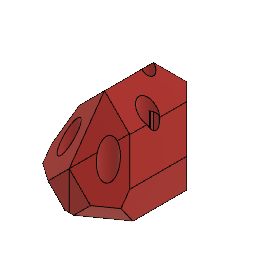
ender_sw_stealth_idler (Autodesk Fusion 360 design; units mm, degrees)
Autodesk Fusion 360 part; units mm, degrees
sketch "Sketch1" plane through (0, 0, 0) normal (0, 0, 1) x (1, 0, 0)
  line L0 (0, 0) -> (-1, 0) construction
  line L1 (-1, 0) -> (-41, 0)
  line L2 (-41, 0) -> (-41, 60)
  line L3 (-41, 60) -> (-1, 60)
  line L4 (-1, 60) -> (-1, 0)
  line L5 (-1, 0) -> (-21, 0) construction
  line L6 (-21, 0) -> (-21, 65.8302) construction
  line L7 (-1, 0) -> (-1, 20) construction
  line L8 (-1, 20) -> (-78.7718, 20) construction
  line L9 (-21, 0) -> (-21, 10) construction
  line L10 (-21, 10) -> (-11, 10) construction
  circle A0 centre (-11, 10) radius 2.55
  circle A1 centre (-11, 30) radius 2.55
  circle A2 centre (-31, 10) radius 2.55
  circle A3 centre (-31, 30) radius 2.55
  line L11 (-21, 20) -> (-21, 30) construction
  line L12 (-16, 35) -> (-26, 35)
  line L13 (-26, 35) -> (-26, 25)
  line L14 (-26, 25) -> (-16, 25)
  line L15 (-16, 25) -> (-16, 35)
  line L16 (-16, 35) -> (-26, 25) construction
  line L17 (-26, 35) -> (-16, 25) construction
  line L18 (-21, 30) -> (-21, 40) construction
  line L19 (-8.75, 46.5) -> (-33.25, 46.5)
  line L20 (-33.25, 46.5) -> (-33.25, 33.5)
  line L21 (-33.25, 33.5) -> (-8.75, 33.5)
  line L22 (-8.75, 33.5) -> (-8.75, 46.5)
  line L23 (-8.75, 46.5) -> (-33.25, 33.5) construction
  line L24 (-33.25, 46.5) -> (-8.75, 33.5) construction
  line L25 (-26, 48) -> (-16, 48)
  line L26 (-16, 48) -> (-16, 45)
  line L27 (-16, 45) -> (-26, 45)
  line L28 (-26, 45) -> (-26, 48)
  line L29 (-26, 48) -> (-16, 45) construction
  line L30 (-16, 48) -> (-26, 45) construction
  circle A4 centre (-21, 40) radius 1.55
  point P0 (-21, 30)
  point P1 (-21, 40)
  point P2 (-21, 46.5)
  dimension "d1" = 1
  dimension "d2" = 40
  dimension "d3" = 60
  dimension "d4" = 20
  dimension "d5" = 20
  dimension "d6" = 10
  dimension "d7" = 10
  dimension "d8" = 5.1
  dimension "d12" = 10
  dimension "d13" = 10
  dimension "d14" = 10
  dimension "d15" = 10
  dimension "d16" = 24.5
  dimension "d17" = 13
  dimension "d18" = 10
  dimension "d19" = 3
  dimension "d30" = 3.1
  constraint coincident L0.start origin
  constraint horizontal L0
  constraint horizontal L1
  constraint vertical L2
  constraint horizontal L3
  constraint vertical L4
  constraint perpendicular L4 L5
  constraint perpendicular L5 L6
  constraint perpendicular L1 L7
  constraint perpendicular L4 L8
  constraint perpendicular L1 L9
  constraint perpendicular L9 L10
  constraint coincident L10.end A0.centre
  constraint symmetric L8 A0 A1
  constraint symmetric L6 A0 A2
  constraint symmetric L6 A1 A3
  constraint coincident L8 L11.start
  constraint coincident L6 L11.start
  constraint perpendicular L8 L11
  constraint horizontal L12
  constraint perpendicular L12 L13
  constraint parallel L12 L14
  constraint parallel L13 L15
  constraint coincident L16 P0
  constraint coincident L17 P0
  constraint coincident P0 L11.end
  constraint perpendicular L12 L18
  constraint horizontal L19
  constraint perpendicular L19 L20
  constraint parallel L19 L21
  constraint parallel L20 L22
  constraint coincident L23 P1
  constraint coincident L24 P1
  constraint coincident P1 L18.end
  constraint horizontal L25
  constraint perpendicular L25 L26
  constraint parallel L25 L27
  constraint parallel L26 L28
  constraint coincident L29 P2
  constraint coincident L30 P2
  constraint midpoint L19 P2
  measures "d1" distance of L0.start L0.end
  measures "d2" distance of L0.end L1.end
  measures "d3" distance of L0.end L3.end
  measures "d4" distance of L0.end L5.end
  measures "d5" distance of L0.end L7.end
  measures "d6" distance of L5.end L9.end
  measures "d7" distance of L9.end L10.end
  measures "d8" diameter of A0
  measures "d12" distance of L11.start P0
  measures "d13" distance of L13.end L14.end
  measures "d14" distance of L12.end L13.end
  measures "d15" distance of P0 P1
  measures "d16" distance of L20.end L21.end
  measures "d17" distance of L19.end L20.end
  measures "d18" distance of L26.end L27.end
  measures "d19" distance of L25.end L26.end
  measures "d30" diameter of A4
extrude "Extrude1" add sketch "Sketch1" along normal blind 45 contours L1 L2 L3 L4 | A0 | A1 | A2 | A3 | L12 L13 L15 L21 | L12 L13 L15 L19 L20 L21 L22 L26 L27 L28 | L13 L14 L15 L21 | L19 L26 L27 L28 | L19 L25 L26 L28 | A4
extrude "Extrude2" cut sketch "Sketch1" along normal up to surface (45 mm away) contours A0 | A1 | A2 | A3 | A4
extrude "Extrude3" cut sketch "Sketch1" along normal blind 32 contours L12 L13 L15 L21 | L12 L13 L15 L19 L20 L21 L22 L26 L27 L28 | L13 L14 L15 L21 | L19 L26 L27 L28 | L19 L25 L26 L28 | A4
sketch "Sketch2" plane through (0, 0, 45) normal (0, 0, 1) x (-1, 0, 0)
  circle A0 centre (31, -30) radius 2.55
  circle A1 centre (31, -10) radius 2.55
  circle A2 centre (11, -30) radius 2.55
  circle A3 centre (11, -10) radius 2.55
  circle A4 centre (21, -40) radius 1.55
  line L0 (1, -60) -> (41, -60)
  line L1 (41, -60) -> (41, 0)
  line L2 (41, 0) -> (1, 0)
  line L3 (1, 0) -> (1, -60)
  circle A5 centre (21, -40) radius 3
  circle A6 centre (31, -30) radius 4.35
  circle A7 centre (11, -30) radius 4.35
  circle A8 centre (31, -10) radius 4.35
  circle A9 centre (11, -10) radius 4.35
  dimension "d31" = 6
  dimension "d32" = 8.7
  dimension "d33" = 8.7
  dimension "d34" = 8.7
  dimension "d35" = 8.7
  constraint concentric A4 A5
  constraint concentric A0 A6
  constraint concentric A2 A7
  constraint concentric A1 A8
  constraint concentric A3 A9
  measures "d31" diameter of A5
  measures "d32" diameter of A6
  measures "d33" diameter of A7
  measures "d34" diameter of A8
  measures "d35" diameter of A9
extrude "Extrude4" cut sketch "Sketch2" against normal up to surface (40 mm away) contours A6 | A7 | A8 | A9
extrude "Extrude5" cut sketch "Sketch2" against normal up to surface (8 mm away) contours A5
ref_plane "WorkPlane1" through (-21, 30, 22.5) normal (-1, 0, 0) x (0, -1, 0)
split_face "SplitFace2" 3 faces at (-20.9253, 54.3305, 45) (-27.6667, 60, 30) (-14.3333, 0, 30) by plane through (-21, 30, 22.5) normal (-1, 0, 0)
chamfer "Chamfer14" distance 17 angle 45 2 edges at (-11, 60, 45) (-31, 60, 45)
chamfer "Chamfer21" distance 20 angle 45 2 edges at (-41, 21.5, 45) (-1, 21.5, 45)
chamfer "Chamfer22" distance 18 angle 45 2 edges at (-31, 0, 35) (-11, 0, 35)
chamfer "Chamfer23" distance 20 angle 45 2 edges at (-41, 60, 12.5) (-1, 60, 12.5)
chamfer "Chamfer24" distance 10 angle 45 2 edges at (-1, 29, 25) (-41, 29, 25)
chamfer "Chamfer25" distance 10 angle 45 2 edges at (-40.7721, 0.1612, 0) (-1.2279, 0.1612, 0)
equation "d3 = endheight"
equation "idlerboxw = 24.5 mm"
equation "idlerboxt = 13 mm"
equation "endheight = 60 mm"
equation "d32 = m5screwhead"
equation "d33 = m5screwhead"
equation "d34 = m5screwhead"
equation "d35 = m5screwhead"
equation "m5screwhead = 8.7 mm"
